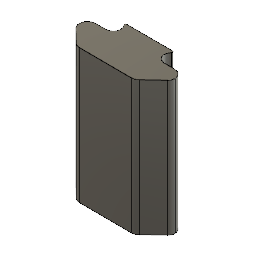
1010RailGuide (Autodesk Fusion 360 design; units mm, degrees)
Autodesk Fusion 360 part; units mm, degrees
sketch "Sketch1" plane through (0, 0, 0) normal (0, 1, 0) x (1, 0, 0)
  circle A0 centre (0, 0) radius 2.605
  line L0 (4.4994, 6.0128) -> (4.4543, -3.0271)
  line L1 (4.4543, -3.0271) -> (-4.5856, -2.982)
  line L2 (-4.5856, -2.982) -> (-4.5404, 6.0579)
  line L3 (-4.5404, 6.0579) -> (4.4994, 6.0128)
  circle A1 centre (-4.3482, 11.5015) radius 1.105
  circle A2 centre (4.3617, 11.4835) radius 1.105
  line L4 (4.3617, 10.3785) -> (10.3577, 10.3785)
  line L5 (4.3617, 12.5885) -> (12.5677, 12.5885)
  circle A3 centre (11.4627, 4.3615) radius 1.105
  line L6 (10.3577, 4.3615) -> (10.3577, 10.3785)
  line L7 (12.5677, 4.3615) -> (12.5677, 12.5885)
  line L8 (-4.3482, 11.5015) -> (-4.3523, 10.3965)
  line L9 (8.5967, 7.0548) -> (4.4841, 2.9422)
  line L10 (8.5967, 7.0548) -> (10.3577, 8.8158)
  line L11 (7.034, 8.6175) -> (4.2894, 6.0138)
  line L12 (-4.3441, 12.6065) -> (-12.5965, 12.6065)
  line L13 (-4.3523, 10.3965) -> (-10.3865, 10.3965)
  circle A4 centre (-11.4915, 4.3915) radius 1.105
  line L14 (-11.4915, 4.3915) -> (-10.3865, 4.3915)
  line L15 (-11.4915, 4.3915) -> (-12.5965, 4.3915)
  line L16 (-12.5965, 4.3915) -> (-12.5965, 12.6065)
  line L17 (-10.3865, 10.3965) -> (-10.3865, 4.3915)
  line L18 (-6.3889, 7.9616) -> (-8.8238, 10.3965)
  line L19 (-7.9516, 6.3989) -> (-10.3865, 8.8338)
  line L20 (-7.9516, 6.3989) -> (-4.5557, 3.003)
  line L21 (-6.3889, 7.9616) -> (-4.3998, 6.0572)
  line L22 (-4.3441, 12.6065) -> (4.3617, 12.5885)
  line L23 (7.034, 8.6175) -> (8.795, 10.3785)
  line L24 (-8.8238, 10.3965) -> (-4.3523, 10.3965)
  line L25 (4.2894, 6.0138) -> (8.795, 10.3785)
  line L26 (8.795, 10.3785) -> (4.3617, 10.3785)
  dimension "d1" = 5.21
  dimension "d4" = 9.04
  dimension "d5" = 9.04
  dimension "d6" = 9.04
  constraint coincident A0.centre origin
  constraint perpendicular L0 L1
  constraint perpendicular L1 L2
  constraint coincident A2 L5.start
  constraint horizontal L4
  constraint horizontal L5
  constraint coincident A1 L12.start
  constraint coincident A1.centre L8.start
  constraint coincident L0 L9.end
  constraint coincident L6 L10.end
  constraint coincident L3 L11.end
  constraint horizontal L12
  constraint horizontal L13
  constraint coincident A4.centre L14.start
  constraint coincident A4 L14.end
  constraint coincident A4 L15.end
  constraint coincident L13 L18.end
  constraint coincident L17 L19.end
  constraint coincident L2 L20.end
  constraint coincident L3 L21.end
  constraint coincident L4 L23.end
  constraint parallel L13 L24
  constraint tangent A2 L26
  measures "d1" diameter of A0
  measures "d4" distance of L0.start L0.end
  measures "d5" distance of L0.end L1.end
  measures "d6" distance of L1.end L2.end
extrude "Extrude3" add sketch "Sketch1" along normal blind 20 contours L11 L23 L25 | L3 A1 A2 L4 L13 L18 L21 L22 L24 L25 L26
fillet "Fillet5" radius 1.23 2 edges at (-8.8238, 10, -10.3965) (8.795, 10, -10.3785)
fillet "Fillet6" radius 1.23 2 edges at (-4.3998, 10, -6.0572) (4.2894, 10, -6.0138)
fillet "Fillet7" radius 0.2 2 edges at (-4.3441, 10, -12.6065) (4.3617, 10, -12.5885)
fillet "Fillet8" radius 1 1 edges at (7.034, 10, -8.6175)
extrude "Extrude1" [suppressed]
sketch "Sketch2" plane through (0.0261, 0, -12.5975) normal (0.00207, 0, -0.999998) x (-0.999998, 0, -0.00207)
  line L0 (4.3702, 20) -> (-4.3356, 20)
  line L1 (-4.3356, 0) -> (4.3702, 0)
  circle A0 centre (-0.0075, 10) radius 3
  line L2 (4.3702, 0) -> (4.3702, 20)
  line L3 (-4.3356, 20) -> (-4.3356, 0)
  dimension "d57" = 6
  measures "d57" diameter of A0
extrude "Extrude2" [suppressed]
fillet "Fillet2" [suppressed]
fillet "Fillet3" [suppressed]
fillet "Fillet4" [suppressed]
fillet "Fillet1" [suppressed]
